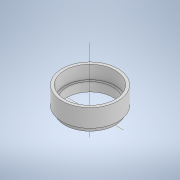
# Autodesk Inventor part: 2020-simulatedFilterWithThreads
Saved by Autodesk Inventor 2020.2 (Build 242310000, 310)
## iProperties
Created: 2020-04-14
Part Number: 2020-simulatedFilterWithThreads
Material: Generic
Document SubType Name: Modeling
Designer: robst
Density: 1 g/cm^3
Appearance: Default
Author: robst
Autodesk Inventor part; units mm, degrees
ref_plane "YZ Plane" through (0, 0, 0) normal (1, 0, 0) x (0, 1, 0)
ref_plane "XZ Plane" through (0, 0, 0) normal (0, 1, 0) x (-1, 0, 0)
ref_plane "XY Plane" through (0, 0, 0) normal (0, 0, 1) x (1, 0, 0)
sketch "Sketch2" plane through (0, 0, 0) normal (0, 0, 1) x (1, 0, 0)
  line L0 (14.2875, 0) -> (14.2875, 2.54)
  line L1 (14.2875, 2.54) -> (15.875, 2.54)
  line L2 (15.875, 2.54) -> (15.875, 12.7)
  line L3 (14.2875, 0) -> (13.0175, 0)
  line L4 (13.0175, 0) -> (13.0175, 5.08)
  line L5 (13.0175, 5.08) -> (14.2875, 5.08)
  line L6 (14.2875, 5.08) -> (14.2875, 12.7)
  line L7 (14.2875, 12.7) -> (15.875, 12.7)
  line L8 (0, -2.54) -> (0, 15.24) projected
  line L9 (-3.175, 0) -> (19.05, 0) projected
  point P0 (0, 0)
  dimension "d8" = 15.875
  dimension "d9" = 14.2875
  dimension "d10" = 2.54
  dimension "d11" = 1.27
  dimension "d12" = 2.54
  dimension "d55" = 7.62
  constraints: 16 end point, 5 perpendicular, 1 collinear, 1 horizontal, 1 parallel, 1 vertical
  measures "d8" distance from line of point (0, 0) L2
  measures "d9" distance from line of point (0, 0) L0
  measures "d10" distance of L0.end L0.start
  measures "d11" distance of L0.start L3.end
  measures "d12" distance of L0.end L5.end
  measures "d55" distance of L5.end L6.end
revolve "Revolution2" add sketch "Sketch2" angle 360 about axis through (0, -10, 0) along (0, 1, 0)
sketch "Sketch4" plane through (0, 9.4283, 0) normal (-1, 0, 0) x (0, 0, 1)
  line L0 (14.2875, 0) -> (14.2875, 20.1694)
  line L1 (14.2875, 20.1694) -> (13.8391, 20.1694)
  line L2 (13.8391, 20.1694) -> (13.8391, 0)
  line L3 (13.8391, 0) -> (14.2875, 0)
  line L4 (0, -4.0339) -> (0, 24.2033) projected
  constraints: 8 end point
sketch "Sketch3" plane through (0, 9.4283, 14.2875) normal (1, 0, 0) x (0, 1, 0)
  line L0 (-0.3529, -0.0308) -> (-0.3025, -0.0308) construction
  line L1 (0.0503, -0.418) -> (-0.0001, -0.5148) construction
  line L2 (-0.6049, -0.5148) -> (-0.6553, -0.418) construction
  line L3 (-0.2521, -0.0308) -> (-0.3025, 0.0661) construction
  line L4 (-0.3025, 0.0661) -> (-0.3529, -0.0308) construction
  line L5 (-0.6049, -0.5148) -> (-0.5545, -0.418) construction
  line L6 (-0.2521, -0.0308) -> (-0.0505, -0.418)
  line L7 (-0.6553, -0.418) -> (-0.5545, -0.418) construction
  arc A0 (-0.6553, -0.418) -> (-0.6049, -0.4486) centre (-0.6049, -0.3918) ccw construction
  line L8 (0.0503, -0.418) -> (-0.0505, -0.418) construction
  line L9 (-0.6049, -0.5148) -> (-0.6049, -0.418) construction
  line L10 (-0.0001, -0.5148) -> (-0.0001, -0.418) construction
  line L11 (-0.3025, 0.0661) -> (-0.3025, -0.0002) construction
  line L12 (-0.6049, -0.4486) -> (-0.0001, -0.4486)
  arc A1 (-0.6049, -0.4486) -> (-0.5545, -0.418) centre (-0.6049, -0.3918) ccw
  line L13 (-0.0505, -0.418) -> (-0.0001, -0.5148) construction
  line L14 (-0.5545, -0.418) -> (-0.3529, -0.0308)
  line L15 (-0.0001, -0.0002) -> (-0.0001, 0.0177)
  line L16 (-0.0001, 0.0177) -> (-0.0001, -0.0002)
  line L17 (-0.0001, -0.0002) -> (0.0334, -0.0002)
  arc A2 (-0.0505, -0.418) -> (-0.0001, -0.4486) centre (-0.0001, -0.3918) ccw
  arc A3 (-0.0001, -0.4486) -> (0.0503, -0.418) centre (-0.0001, -0.3918) ccw construction
  arc A4 (-0.3025, -0.0002) -> (-0.3529, -0.0308) centre (-0.3025, -0.057) ccw
  arc A5 (-0.2521, -0.0308) -> (-0.3025, -0.0002) centre (-0.3025, -0.057) ccw
  line L18 (-0.3025, -0.0002) -> (-0.3025, -0.0308) construction
  line L19 (-0.3025, -0.0308) -> (-0.2521, -0.0308) construction
  dimension "d18" = 55
  dimension "d19" = 0.0968
  dimension "d20" = 0.0968
  dimension "Sketch3_ThreadOffset" = 0
  dimension "Sketch3_MajorRadius" = 0.4484
  dimension "d23" = 0.6048
  dimension "Sketch3_MinorRadius" = 0
  constraints: 40 end point, 12 point on circle, 10 parallel, 8 tangent, 6 centre point, 6 collinear, 2 midpoint, 2 point on line, 1 horizontal, 1 perpendicular, 3 other
  measures "d18" angle of L6 L14
  measures "d19" distance of L3.end L0.end
  measures "d20" distance of L1.end L10.end
  measures "Sketch3_ThreadOffset" distance between parallel lines of L15 L10
  measures "Sketch3_MajorRadius" distance from line of L12 L15.start
  measures "d23" distance from line of L1.end L9
  measures "Sketch3_MinorRadius" distance edge to line of A5 L17
sketch "Sketch6" plane through (0, 0, 0) normal (-1, 0, 0) x (0, 0, 1)
  line L0 (14.2875, 0) -> (14.2875, 6.8883)
  line L1 (14.2875, 6.8883) -> (13.8391, 6.8883)
  line L2 (13.8391, 6.8883) -> (13.8391, 0)
  line L3 (13.8391, 0) -> (14.2875, 0)
  line L4 (0, -1.3777) -> (0, 8.2659) projected
  constraints: 8 end point
sketch "Sketch7" plane through (0, 0, 0) normal (-1, 0, 0) x (0, 0, 1)
  line L0 (14.2875, 0) -> (14.2875, 6.8883)
  line L1 (14.2875, 6.8883) -> (13.8391, 6.8883)
  line L2 (13.8391, 6.8883) -> (13.8391, 0)
  line L3 (13.8391, 0) -> (14.2875, 0)
  line L4 (0, -1.3777) -> (0, 8.2659) projected
  constraints: 8 end point
sketch "Sketch5" plane through (0, 0, 0) normal (1, 0, 0) x (0, 1, 0)
  line L0 (-0.3529, -13.8698) -> (-0.3025, -13.8698) construction
  line L1 (0.0503, -14.2571) -> (-0.0001, -14.3539) construction
  line L2 (-0.6049, -14.3539) -> (-0.6553, -14.2571) construction
  line L3 (-0.2521, -13.8698) -> (-0.3025, -13.773) construction
  line L4 (-0.3025, -13.773) -> (-0.3529, -13.8698) construction
  line L5 (-0.6049, -14.3539) -> (-0.5545, -14.2571) construction
  line L6 (-0.2521, -13.8698) -> (-0.0505, -14.2571)
  line L7 (-0.6553, -14.2571) -> (-0.5545, -14.2571) construction
  arc A0 (-0.6553, -14.2571) -> (-0.6049, -14.2877) centre (-0.6049, -14.2309) ccw construction
  line L8 (0.0503, -14.2571) -> (-0.0505, -14.2571) construction
  line L9 (-0.6049, -14.3539) -> (-0.6049, -14.2571) construction
  line L10 (-0.0001, -14.3539) -> (-0.0001, -14.2571) construction
  line L11 (-0.3025, -13.773) -> (-0.3025, -13.8393) construction
  line L12 (-0.6049, -14.2877) -> (-0.0001, -14.2877)
  arc A1 (-0.6049, -14.2877) -> (-0.5545, -14.2571) centre (-0.6049, -14.2309) ccw
  line L13 (-0.0505, -14.2571) -> (-0.0001, -14.3539) construction
  line L14 (-0.5545, -14.2571) -> (-0.3529, -13.8698)
  line L15 (-0.0001, -0.0002) -> (-0.0001, 0.0177)
  line L16 (-0.0001, 0.0177) -> (-0.0001, -0.0002)
  line L17 (-0.0001, -0.0002) -> (0.0334, -0.0002)
  arc A2 (-0.0505, -14.2571) -> (-0.0001, -14.2877) centre (-0.0001, -14.2309) ccw
  arc A3 (-0.0001, -14.2877) -> (0.0503, -14.2571) centre (-0.0001, -14.2309) ccw construction
  arc A4 (-0.3025, -13.8393) -> (-0.3529, -13.8698) centre (-0.3025, -13.8961) ccw
  arc A5 (-0.2521, -13.8698) -> (-0.3025, -13.8393) centre (-0.3025, -13.8961) ccw
  line L18 (-0.3025, -13.8393) -> (-0.3025, -13.8698) construction
  line L19 (-0.3025, -13.8698) -> (-0.2521, -13.8698) construction
  dimension "d36" = 55
  dimension "d37" = 0.0968
  dimension "d38" = 0.0968
  dimension "Sketch5_ThreadOffset" = 0
  dimension "Sketch5_MajorRadius" = 14.2875
  dimension "d41" = 0.6048
  dimension "Sketch5_MinorRadius" = 13.8391
  constraints: 40 end point, 12 point on circle, 10 parallel, 8 tangent, 6 centre point, 6 collinear, 2 midpoint, 2 point on line, 1 horizontal, 1 perpendicular, 3 other
  measures "d36" angle of L6 L14
  measures "d37" distance of L3.end L0.end
  measures "d38" distance of L1.end L10.end
  measures "Sketch5_ThreadOffset" distance between parallel lines of L15 L10
  measures "Sketch5_MajorRadius" distance from line of L12 L15.start
  measures "d41" distance from line of L1.end L9
  measures "Sketch5_MinorRadius" distance edge to line of A5 L17
equation "\"d18\" = d25"
equation "\"d19\" = 0.160083 * Sketch3_Pitch"
equation "\"d20\" = 0.160083 * Sketch3_Pitch"
equation "\"d23\" = Sketch3_Pitch"
equation "\"d36\" = d43"
equation "\"d37\" = 0.160083 * Sketch5_Pitch"
equation "\"d38\" = 0.160083 * Sketch5_Pitch"
equation "\"d41\" = Sketch5_Pitch"
equation "\"d25\" = 55deg"
equation "\"Sketch3_Pitch\" = 0.60476"
equation "\"d43\" = 55deg"
equation "\"Sketch5_Pitch\" = 0.60476"
body "Solid2"
body "Solid3"
body "Solid4"
